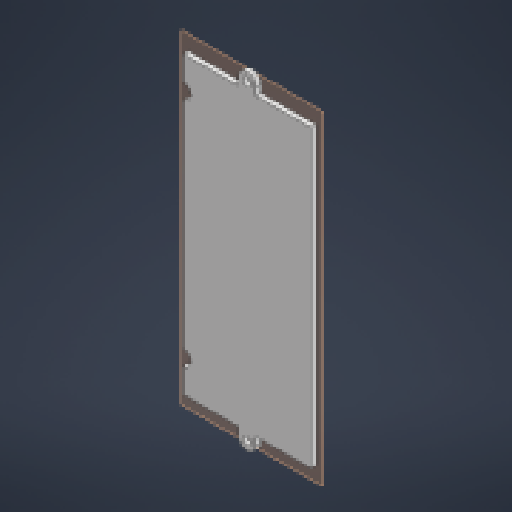
# Autodesk Inventor part: fixture
Saved by Autodesk Inventor 2024.3 (Build 283343000, 343)
## iProperties
Created: 2025-08-11
Part Number: fixture
Material: Generic
Document SubType Name: Modeling
Designer: giuseppe
Density: 1 g/cm^3
Appearance: Default
Author: giuseppe
Autodesk Inventor part; units mm, degrees
ref_plane "YZ Plane" through (0, 0, 0) normal (1, 0, 0) x (0, 1, 0)
ref_plane "XZ Plane" through (0, 0, 0) normal (0, 1, 0) x (-1, 0, 0)
ref_plane "XY Plane" through (0, 0, 0) normal (0, 0, 1) x (1, 0, 0)
ref_plane "Work Plane1" through (0, 0, 5) normal (0, 0, 1) x (1, 0, 0)
sketch "Sketch1" plane through (0, 0, 5) normal (0, 0, 1) x (1, 0, 0)
  line L0 (-17, 38.2524) -> (2, 47.75) construction
  line L1 (2, 47.75) -> (2, 41.6027) construction
  line L2 (2, 41.6027) -> (17, 44.2476) construction
  line L3 (17, 44.2476) -> (-2, 34.75) construction
  line L4 (-2, 34.75) -> (-2, 40.8973) construction
  line L5 (-2, 40.8973) -> (-17, 38.2524) construction
  line L6 (-17, 21.7524) -> (2, 31.25) construction
  line L7 (2, 31.25) -> (2, 25.1027) construction
  line L8 (2, 25.1027) -> (17, 27.7476) construction
  line L9 (17, 27.7476) -> (-2, 18.25) construction
  line L10 (-2, 18.25) -> (-2, 24.3973) construction
  line L11 (-2, 24.3973) -> (-17, 21.7524) construction
  line L12 (-17, 5.2524) -> (2, 14.75) construction
  line L13 (2, 14.75) -> (2, 8.6027) construction
  line L14 (2, 8.6027) -> (17, 11.2476) construction
  line L15 (17, 11.2476) -> (-2, 1.75) construction
  line L16 (-2, 1.75) -> (-2, 7.8973) construction
  line L17 (-2, 7.8973) -> (-17, 5.2524) construction
  line L18 (-17, -11.2476) -> (2, -1.75) construction
  line L19 (2, -1.75) -> (2, -7.8973) construction
  line L20 (2, -7.8973) -> (17, -5.2524) construction
  line L21 (17, -5.2524) -> (-2, -14.75) construction
  line L22 (-2, -14.75) -> (-2, -8.6027) construction
  line L23 (-2, -8.6027) -> (-17, -11.2476) construction
  line L24 (-17, -27.7476) -> (2, -18.25) construction
  line L25 (2, -18.25) -> (2, -24.3973) construction
  line L26 (2, -24.3973) -> (17, -21.7524) construction
  line L27 (17, -21.7524) -> (-2, -31.25) construction
  line L28 (-2, -31.25) -> (-2, -25.1027) construction
  line L29 (-2, -25.1027) -> (-17, -27.7476) construction
  line L30 (-17, -44.2476) -> (2, -34.75) construction
  line L31 (2, -34.75) -> (2, -40.8973) construction
  line L32 (2, -40.8973) -> (17, -38.2524) construction
  line L33 (17, -38.2524) -> (-2, -47.75) construction
  line L34 (-2, -47.75) -> (-2, -41.6027) construction
  line L35 (-2, -41.6027) -> (-17, -44.2476) construction
  line L36 (25, 57.75) -> (25, -57.75) construction
  line L37 (-25, 57.75) -> (25, 57.75) construction
  line L38 (-25, -57.75) -> (-25, 57.75) construction
  line L39 (25, -57.75) -> (-25, -57.75) construction
  line L40 (-25, 57.75) -> (25, 57.75)
  line L41 (25, 57.75) -> (25, -57.75)
  line L42 (25, -57.75) -> (-25, -57.75)
  line L43 (-25, -57.75) -> (-25, 57.75)
  point P0 (0, 0)
  constraints: 8 end point, 2 parallel, 1 horizontal, 1 perpendicular
extrude "Extrusion1" add sketch "Sketch1" along normal blind 2
sketch "Sketch2" plane through (0, 0, 5) normal (0, 0, -1) x (-1, 0, 0)
  line L0 (2, -8.6027) -> (2, -14.75) construction
  line L1 (2, -14.75) -> (-17, -5.2524) construction
  line L2 (-17, -5.2524) -> (-2, -7.8973) construction
  line L3 (-2, -7.8973) -> (-2, -1.75) construction
  line L4 (-2, -1.75) -> (17, -11.2476) construction
  line L5 (17, -11.2476) -> (2, -8.6027) construction
  line L6 (2, 40.8973) -> (2, 34.75) construction
  line L7 (2, 34.75) -> (-17, 44.2476) construction
  line L8 (-17, 44.2476) -> (-2, 41.6027) construction
  line L9 (-2, 41.6027) -> (-2, 47.75) construction
  line L10 (-2, 47.75) -> (17, 38.2524) construction
  line L11 (17, 38.2524) -> (2, 40.8973) construction
  line L12 (2, -25.1027) -> (2, -31.25) construction
  line L13 (2, -31.25) -> (-17, -21.7524) construction
  line L14 (-17, -21.7524) -> (-2, -24.3973) construction
  line L15 (-2, -24.3973) -> (-2, -18.25) construction
  line L16 (-2, -18.25) -> (17, -27.7476) construction
  line L17 (17, -27.7476) -> (2, -25.1027) construction
  line L18 (2, 7.8973) -> (2, 1.75) construction
  line L19 (2, 1.75) -> (-17, 11.2476) construction
  line L20 (-17, 11.2476) -> (-2, 8.6027) construction
  line L21 (-2, 8.6027) -> (-2, 14.75) construction
  line L22 (-2, 14.75) -> (17, 5.2524) construction
  line L23 (17, 5.2524) -> (2, 7.8973) construction
  line L24 (2, 24.3973) -> (2, 18.25) construction
  line L25 (2, 18.25) -> (-17, 27.7476) construction
  line L26 (-17, 27.7476) -> (-2, 25.1027) construction
  line L27 (-2, 25.1027) -> (-2, 31.25) construction
  line L28 (-2, 31.25) -> (17, 21.7524) construction
  line L29 (17, 21.7524) -> (2, 24.3973) construction
  line L30 (2, -41.6027) -> (2, -47.75) construction
  line L31 (2, -47.75) -> (-17, -38.2524) construction
  line L32 (-17, -38.2524) -> (-2, -40.8973) construction
  line L33 (-2, -40.8973) -> (-2, -34.75) construction
  line L34 (-2, -34.75) -> (17, -44.2476) construction
  line L35 (17, -44.2476) -> (2, -41.6027) construction
  line L36 (-25, 57.75) -> (-25, -57.75) construction
  line L37 (-25, -57.75) -> (25, -57.75) construction
  line L38 (25, -57.75) -> (25, 57.75) construction
  line L39 (25, 57.75) -> (-25, 57.75) construction
  line L40 (-20, 33.7) -> (20, 33.7)
  line L41 (20, 33.7) -> (20, 32.3)
  line L42 (20, 32.3) -> (-20, 32.3)
  line L43 (-20, 32.3) -> (-20, 33.7)
  line L44 (-2, 31.25) -> (2, 31.25) construction
  line L45 (2, 31.25) -> (2, 34.75) construction
  line L46 (2, 34.75) -> (-2, 34.75) construction
  line L47 (-2, 34.75) -> (-2, 31.25) construction
  point P0 (0, 0)
  point P1 (-20, 33)
  point P2 (20, 33)
  point P3 (2, 33)
  dimension "d2" = 5
  dimension "d3" = 5
  dimension "d4" = 1.4
  dimension "d7" = 1.05
  dimension "d8" = 6.1474
  constraints: 16 end point, 4 parallel, 3 midpoint, 2 horizontal, 2 perpendicular, 1 horizontal alignment
  measures "d2" distance from line of L36 point (-20, 33)
  measures "d3" distance from line of L38 point (20, 33)
  measures "d4" distance of L42.end L40.start
  measures "d7" distance from line of L40 L6.end
  measures "d8" distance of L6.end L6.start
extrude "Extrusion2" add sketch "Sketch2" along normal blind 5
sketch "Sketch3" plane through (0, 0, 5) normal (0, 0, -1) x (-1, 0, 0)
  line L0 (2, -8.6027) -> (2, -14.75) construction
  line L1 (2, -14.75) -> (-17, -5.2524) construction
  line L2 (-17, -5.2524) -> (-2, -7.8973) construction
  line L3 (-2, -7.8973) -> (-2, -1.75) construction
  line L4 (-2, -1.75) -> (17, -11.2476) construction
  line L5 (17, -11.2476) -> (2, -8.6027) construction
  line L6 (2, 40.8973) -> (2, 34.75) construction
  line L7 (2, 34.75) -> (-17, 44.2476) construction
  line L8 (-17, 44.2476) -> (-2, 41.6027) construction
  line L9 (-2, 41.6027) -> (-2, 47.75) construction
  line L10 (-2, 47.75) -> (17, 38.2524) construction
  line L11 (17, 38.2524) -> (2, 40.8973) construction
  line L12 (2, -25.1027) -> (2, -31.25) construction
  line L13 (2, -31.25) -> (-17, -21.7524) construction
  line L14 (-17, -21.7524) -> (-2, -24.3973) construction
  line L15 (-2, -24.3973) -> (-2, -18.25) construction
  line L16 (-2, -18.25) -> (17, -27.7476) construction
  line L17 (17, -27.7476) -> (2, -25.1027) construction
  line L18 (2, 7.8973) -> (2, 1.75) construction
  line L19 (2, 1.75) -> (-17, 11.2476) construction
  line L20 (-17, 11.2476) -> (-2, 8.6027) construction
  line L21 (-2, 8.6027) -> (-2, 14.75) construction
  line L22 (-2, 14.75) -> (17, 5.2524) construction
  line L23 (17, 5.2524) -> (2, 7.8973) construction
  line L24 (2, 24.3973) -> (2, 18.25) construction
  line L25 (2, 18.25) -> (-17, 27.7476) construction
  line L26 (-17, 27.7476) -> (-2, 25.1027) construction
  line L27 (-2, 25.1027) -> (-2, 31.25) construction
  line L28 (-2, 31.25) -> (17, 21.7524) construction
  line L29 (17, 21.7524) -> (2, 24.3973) construction
  line L30 (2, -41.6027) -> (2, -47.75) construction
  line L31 (2, -47.75) -> (-17, -38.2524) construction
  line L32 (-17, -38.2524) -> (-2, -40.8973) construction
  line L33 (-2, -40.8973) -> (-2, -34.75) construction
  line L34 (-2, -34.75) -> (17, -44.2476) construction
  line L35 (17, -44.2476) -> (2, -41.6027) construction
  line L36 (-25, 57.75) -> (-25, -57.75) construction
  line L37 (-25, -57.75) -> (25, -57.75) construction
  line L38 (25, -57.75) -> (25, 57.75) construction
  line L39 (25, 57.75) -> (-25, 57.75) construction
  line L40 (2, 18.25) -> (-2, 18.25) construction
  line L41 (-2, 18.25) -> (-2, 14.75) construction
  line L42 (-2, 14.75) -> (2, 14.75) construction
  line L43 (2, 14.75) -> (2, 18.25) construction
  line L44 (-2, -1.75) -> (2, -1.75) construction
  line L45 (2, -1.75) -> (2, 1.75) construction
  line L46 (2, 1.75) -> (-2, 1.75) construction
  line L47 (-2, 1.75) -> (-2, -1.75) construction
  line L48 (2, -14.75) -> (-2, -14.75) construction
  line L49 (-2, -14.75) -> (-2, -18.25) construction
  line L50 (-2, -18.25) -> (2, -18.25) construction
  line L51 (2, -18.25) -> (2, -14.75) construction
  line L52 (2, -31.25) -> (-2, -31.25) construction
  line L53 (-2, -31.25) -> (-2, -34.75) construction
  line L54 (-2, -34.75) -> (2, -34.75) construction
  line L55 (2, -34.75) -> (2, -31.25) construction
  point P0 (0, 0)
  point P1 (0, -33)
  point P2 (-2, -33)
  point P3 (0, -31.25)
  point P4 (0, -16.5)
  point P5 (0, 0)
  point P6 (0, 16.5)
  point P7 (0, 18.25)
  point P8 (0, 1.75)
  point P9 (0, -14.75)
  point P10 (-2, 16.5)
  point P11 (-2, 0)
  point P12 (-2, -16.5)
  constraints: 32 end point, 8 midpoint, 8 parallel, 4 horizontal, 4 horizontal alignment, 4 perpendicular, 4 vertical alignment
pattern_sketch "Sketch Driven Pattern1" of "Extrusion2" from (0, 33, 5) copies at (0, -33, 5) at (0, -16.5, 5) at (0, 0, 5) at (0, 16.5, 5)
sketch "Sketch4" plane through (0, 0, 7) normal (0, 0, 1) x (1, 0, 0)
  circle A0 centre (0, -60.75) radius 1.65
  line L0 (3.5, -60.75) -> (-3.5, -60.75)
  line L1 (-3.5, -60.75) -> (-3.5, -57.75)
  line L2 (-3.5, -57.75) -> (3.5, -57.75)
  line L3 (3.5, -57.75) -> (3.5, -60.75)
  arc A1 (-3.5, -60.75) -> (3.5, -60.75) centre (0, -60.75) ccw
  line L4 (-25, -57.75) -> (25, -57.75) projected
  point P0 (0, 0)
  point P1 (0, -57.75)
  dimension "d9" = 7
  dimension "d10" = 3.3
  dimension "d11" = 3
  constraints: 9 end point, 2 centre point, 2 coincident, 2 midpoint, 2 parallel, 2 point on circle, 1 collinear, 1 horizontal, 1 perpendicular, 1 vertical alignment
  measures "d9" distance of L0.start L0.end
  measures "d10" diameter of A0
  measures "d11" distance of L0.end L1.end
extrude "Extrusion3" add sketch "Sketch4" against normal up to surface (2 mm away) contours L0 A1 A0 | A0 L0 L1 L2 L3
mirror "Mirror1" about plane through (0, 0, 0) normal (0, 1, 0) of "Extrusion3"
sketch "Sketch5" plane through (0, 0, 5) normal (0, 0, -1) x (-1, 0, 0)
  line L0 (25, 57.75) -> (25, -57.75) projected
  arc A0 (25, 48.0971) -> (25, 42.0971) centre (25, 45.0971) ccw
  line L1 (25, 48.0971) -> (25, 42.0971)
  point P0 (0, 0)
  dimension "d14" = 3
  constraints: 2 end point, 2 point on circle, 2 point on line, 1 centre point, 1 collinear
  measures "d14" radius of A0
extrude "Extrusion4" cut sketch "Sketch5" against normal blind 10
mirror "Mirror2" about plane through (0, 0, 0) normal (0, 1, 0) of "Extrusion4"
body "Solid1"
